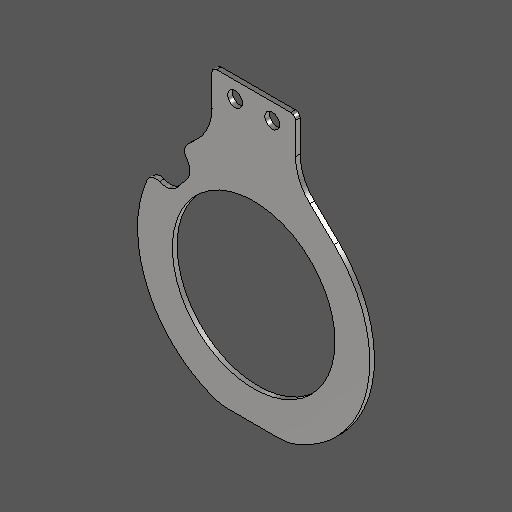
# Autodesk Inventor part: probe-gate
Saved by Autodesk Inventor 2025 (Build 290162000, 162)
## iProperties
Created: 2024-05-15
Part Number: probe-gate
Material: Stainless Steel
Document SubType Name: Modeling
Designer: queezz
Density: 8 g/cm^3
Appearance: Semi-Polished
Author: queezz
Autodesk Inventor part; units mm, degrees
ref_plane "YZ Plane" through (0, 0, 0) normal (1, 0, 0) x (0, 1, 0)
ref_plane "XZ Plane" through (0, 0, 0) normal (0, 1, 0) x (-1, 0, 0)
ref_plane "XY Plane" through (0, 0, 0) normal (0, 0, 1) x (1, 0, 0)
sketch "Sketch1" plane through (0, 0, 0) normal (0, 0, 1) x (1, 0, 0)
  line L0 (-9, 26) -> (-9, 38)
  line L1 (-9, 38) -> (9, 38)
  line L2 (9, 38) -> (9, 26)
  line L3 (9, 26) -> (17.2958, 18.0514)
  line L4 (-9, 26) -> (-17.2958, 18.0514)
  arc A0 (-17.2958, 18.0514) -> (17.2958, 18.0514) centre (0, 0) ccw
  line L5 (-17.2958, 18.0514) -> (17.2958, 18.0514) construction
  line L6 (-9, 26) -> (9, 26) construction
  circle A1 centre (0, 0) radius 17.5
  point P0 (0, 38)
  dimension "d1" = 38
  dimension "d2" = 18
  dimension "d3" = 50
  dimension "d5" = 35
  dimension "d15" = 12
  constraints: 14 end point, 2 centre point, 2 coincident, 2 horizontal, 2 perpendicular, 2 point on circle, 1 midpoint, 1 tangent, 1 vertical, 1 vertical alignment
  measures "d1" distance from line of A0.centre L1
  measures "d2" distance of L0.end L1.end
  measures "d3" diameter of A0
  measures "d5" diameter of A1
  measures "d15" distance between parallel lines of L1 L6
extrude "Extrusion1" add sketch "Sketch1" along normal blind 1
fillet "Fillet1" radius 10 2 edges at (9, 26, 0.5) (-9, 26, 0.5)
fillet "Fillet2" radius 1 2 edges at (9, 38, 0.5) (-9, 38, 0.5)
sketch "Sketch2" plane through (0, 0, 1) normal (0, 0, 1) x (1, 0, 0)
  circle A0 centre (-4, 34.5) radius 1.6
  circle A1 centre (4, 34.5) radius 1.6
  line L0 (-4, 34.5) -> (4, 34.5) construction
  line L1 (8, 38) -> (-8, 38) construction
  point P0 (0, 0)
  point P1 (0, 34.5)
  dimension "d10" = 3.5
  dimension "d11" = 3.2
  dimension "d12" = 8
  constraints: 2 centre point, 2 end point, 1 equal radius, 1 horizontal, 1 midpoint, 1 vertical alignment
  measures "d10" distance between parallel lines of L1 L0
  measures "d11" diameter of A1
  measures "d12" distance of L0.start L0.end
extrude "Extrusion2" cut sketch "Sketch2" against normal through all
sketch "Sketch3" plane through (0, 0, 0) normal (0, 0, 1) x (1, 0, 0)
  line L0 (-15, -30) -> (15, -30)
  line L1 (15, -30) -> (15, -24)
  line L2 (15, -24) -> (-15, -24)
  line L3 (-15, -24) -> (-15, -30)
  point P0 (0, 0)
  point P1 (0, -24)
  dimension "d16" = 24
  dimension "d17" = 6
  dimension "d18" = 30
  constraints: 8 end point, 2 parallel, 1 horizontal, 1 midpoint, 1 perpendicular, 1 vertical alignment
  measures "d16" distance from line of point (0, 0) L2
  measures "d17" distance of L0.end L1.end
  measures "d18" distance of L1.end L2.end
extrude "Trim" cut sketch "Sketch3" along normal through all
fillet "Fillet3" radius 10 2 edges at (7, -24, 0.5) (-7, -24, 0.5)
sketch "Sketch4" plane through (0, 0, 1) normal (0, 0, 1) x (1, 0, 0)
  line L0 (-18.002, 15.1055) -> (18.002, -15.1055) construction
  line L1 (0, 0) -> (14.5661, 0) construction
  arc A0 (-17.0012, 16.2238) -> (-18.9295, 13.9256) centre (0, 0) ccw construction
  arc A1 (-19.3524, 18.4675) -> (-21.5474, 15.8515) centre (0, 0) ccw
  arc A2 (-14.6499, 13.9801) -> (-16.3116, 11.9998) centre (0, 0) ccw
  arc A3 (-14.6499, 13.9801) -> (-19.3524, 18.4675) centre (-17.0012, 16.2238) ccw
  arc A4 (-21.5474, 15.8515) -> (-16.3116, 11.9998) centre (-18.9295, 13.9256) ccw
  dimension "d24" = 40
  dimension "d28" = 47
  dimension "d29" = 6.5
  dimension "d30" = 3
  constraints: 11 point on circle, 5 centre point, 4 end point, 4 tangent, 2 coincident, 1 horizontal, 1 midpoint
  measures "d24" angle of L0 L1
  measures "d28" diameter of A0
  measures "d29" diameter of A3
  measures "d30" distance of A0.end A0.start
extrude "Extrusion4" cut sketch "Sketch4" against normal through all
fillet "Fillet5" radius 2 2 edges at (-15.9823, 19.31, 0.5) (-21.7544, 12.3186, 0.5)
body "Solid1"
